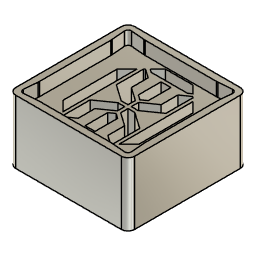
teenage_engineering_display (Autodesk Fusion 360 design; units mm, degrees)
Autodesk Fusion 360 part; units mm, degrees
sketch "8x8_led_matrix_display" plane through (0, 0, 0) normal (0, 0, 1) x (1, 0, 0)
  circle A0 centre (-14, 14) radius 1.5
  circle A1 centre (-10, 14) radius 1.5
  circle A2 centre (-6, 14) radius 1.5
  circle A3 centre (-2, 14) radius 1.5
  circle A4 centre (2, 14) radius 1.5
  circle A5 centre (6, 14) radius 1.5
  circle A6 centre (10, 14) radius 1.5
  circle A7 centre (14, 14) radius 1.5
  circle A8 centre (-14, 10) radius 1.5
  circle A9 centre (-10, 10) radius 1.5
  circle A10 centre (-6, 10) radius 1.5
  circle A11 centre (-2, 10) radius 1.5
  circle A12 centre (2, 10) radius 1.5
  circle A13 centre (6, 10) radius 1.5
  circle A14 centre (10, 10) radius 1.5
  circle A15 centre (14, 10) radius 1.5
  circle A16 centre (-14, 6) radius 1.5
  circle A17 centre (-10, 6) radius 1.5
  circle A18 centre (-6, 6) radius 1.5
  circle A19 centre (-2, 6) radius 1.5
  circle A20 centre (2, 6) radius 1.5
  circle A21 centre (6, 6) radius 1.5
  circle A22 centre (10, 6) radius 1.5
  circle A23 centre (14, 6) radius 1.5
  circle A24 centre (-14, 2) radius 1.5
  circle A25 centre (-10, 2) radius 1.5
  circle A26 centre (-6, 2) radius 1.5
  circle A27 centre (-2, 2) radius 1.5
  circle A28 centre (2, 2) radius 1.5
  circle A29 centre (6, 2) radius 1.5
  circle A30 centre (10, 2) radius 1.5
  circle A31 centre (14, 2) radius 1.5
  circle A32 centre (-14, -2) radius 1.5
  circle A33 centre (-10, -2) radius 1.5
  circle A34 centre (-6, -2) radius 1.5
  circle A35 centre (-2, -2) radius 1.5
  circle A36 centre (2, -2) radius 1.5
  circle A37 centre (6, -2) radius 1.5
  circle A38 centre (10, -2) radius 1.5
  circle A39 centre (14, -2) radius 1.5
  circle A40 centre (-14, -6) radius 1.5
  circle A41 centre (-10, -6) radius 1.5
  circle A42 centre (-6, -6) radius 1.5
  circle A43 centre (-2, -6) radius 1.5
  circle A44 centre (2, -6) radius 1.5
  circle A45 centre (6, -6) radius 1.5
  circle A46 centre (10, -6) radius 1.5
  circle A47 centre (14, -6) radius 1.5
  circle A48 centre (-14, -10) radius 1.5
  circle A49 centre (-10, -10) radius 1.5
  circle A50 centre (-6, -10) radius 1.5
  circle A51 centre (-2, -10) radius 1.5
  circle A52 centre (2, -10) radius 1.5
  circle A53 centre (6, -10) radius 1.5
  circle A54 centre (10, -10) radius 1.5
  circle A55 centre (14, -10) radius 1.5
  circle A56 centre (-14, -14) radius 1.5
  circle A57 centre (-10, -14) radius 1.5
  circle A58 centre (-6, -14) radius 1.5
  circle A59 centre (-2, -14) radius 1.5
  circle A60 centre (2, -14) radius 1.5
  circle A61 centre (6, -14) radius 1.5
  circle A62 centre (10, -14) radius 1.5
  circle A63 centre (14, -14) radius 1.5
  line L0 (16, -16) -> (-16, -16)
  line L1 (-16, -16) -> (-16, 16)
  line L2 (-16, 16) -> (16, 16)
  line L3 (16, 16) -> (16, -16)
  line L4 (16, -16) -> (-16, 16) construction
  line L5 (-16, -16) -> (16, 16) construction
  line L6 (18, -18) -> (-18, -18)
  line L7 (-18, -18) -> (-18, 18)
  line L8 (-18, 18) -> (18, 18)
  line L9 (18, 18) -> (18, -18)
  dimension "d1" = 3
  dimension "d2" = 14
  dimension "d3" = 14
  dimension "d6" = 28
  dimension "d7" = -28
  dimension "d8" = 32
  dimension "d9" = 32
  dimension "d33" = -2
  constraint horizontal L0
  constraint perpendicular L0 L1
  constraint parallel L0 L2
  constraint parallel L1 L3
  constraint coincident L4 origin
  constraint coincident L5 origin
  measures "d1" diameter of A0
  measures "d2" horizontal distance of origin A0.centre
  measures "d3" vertical distance of origin A0.centre
  measures "d8" distance of L1.end L2.end
  measures "d9" distance of L0.end L1.end
sketch "segments" plane through (0, 0, 0) normal (0, 0, 1) x (1, 0, 0)
  line L0 (0, 0) -> (-16, 0)
  line L1 (-16, 0) -> (-16, 16)
  line L2 (-16, 16) -> (0, 16)
  line L3 (0, 16) -> (0, 0)
  line L4 (-11.5, 0) -> (-11.5, 8.1712)
  line L5 (-11.5, 8.1712) -> (-8.5, 11.1712)
  line L6 (-8.5, 11.1712) -> (-8.5, 0)
  line L7 (-7.5, 12.1712) -> (-7.5, 3.961)
  line L8 (-7.5, 3.961) -> (-2.5572, 0.5)
  line L9 (-2.5572, 0.5) -> (-0.5, 0.5)
  line L10 (-0.5, 0.5) -> (-0.5, 2.7218)
  line L11 (-0.5, 2.7218) -> (-4.5, 5.5227)
  line L12 (-4.5, 5.5227) -> (-4.5, 10.5993)
  line L13 (-4.5, 10.5993) -> (-7.189, 12.4822)
  line L14 (-7.189, 12.4822) -> (-7.5, 12.1712)
  line L15 (0, 11.5) -> (-1.5, 11.5)
  line L16 (-1.5, 11.5) -> (-1.5, 4.6428)
  line L17 (-1.5, 4.6428) -> (0, 3.5925)
  line L18 (0, 15.5) -> (-4.1712, 15.5)
  line L19 (-4.1712, 15.5) -> (-6.471, 13.2002)
  line L20 (-6.471, 13.2002) -> (-5.471, 12.5)
  line L21 (-5.471, 12.5) -> (0, 12.5)
  dimension "d10" = 16
  dimension "d11" = 16
  dimension "d12" = 3
  dimension "d13" = 8.5
  dimension "d14" = 3
  dimension "d15" = 3
  dimension "d16" = 0.5
  dimension "d17" = 0.5
  dimension "d18" = 1
  dimension "d19" = 1.5
  dimension "d20" = 11.5
  dimension "d21" = 1
  dimension "d22" = 3
  dimension "d23" = 15.5
  dimension "d24" = 1
  dimension "d25" = 45
  dimension "d26" = 125
  constraint horizontal L0
  constraint vertical L1
  constraint horizontal L2
  constraint vertical L3
  constraint coincident L0.start L3.end
  constraint coincident L0 L4.start
  constraint perpendicular L0 L4
  constraint coincident L0 L6.end
  constraint perpendicular L0 L6
  constraint parallel L6 L7
  constraint perpendicular L6 L9
  constraint perpendicular L9 L10
  constraint parallel L8 L11
  constraint perpendicular L9 L12
  constraint collinear L5 L14
  constraint coincident L3 L15.start
  constraint perpendicular L3 L15
  constraint perpendicular L15 L16
  constraint coincident L3 L17.end
  constraint parallel L11 L17
  constraint coincident L3 L18.start
  constraint perpendicular L3 L18
  constraint coincident L3 L21.end
  constraint perpendicular L3 L21
  constraint parallel L13 L20
  constraint collinear L14 L19
  constraint parallel L11 L13
  measures "d10" distance of L0.start L0.end
  measures "d11" distance of L0.start L2.end
  measures "d12" distance of L4 L6
  measures "d13" distance of L3 L6
  measures "d14" distance of L7 L12
  measures "d15" distance of L8 L11
  measures "d16" distance of L3 L10
  measures "d17" distance of L0 L9
  measures "d18" distance of L6 L7
  measures "d19" distance of L3 L16
  measures "d20" distance of L0 L15
  measures "d21" distance of L11 L17
  measures "d22" distance of L18 L21
  measures "d23" distance of L0 L18
  measures "d24" distance of L13 L20
  measures "d25" angle of L5 L6
  measures "d26" angle of L12 L13
extrude "Extrude1" add sketch "segments" along normal blind 15 contours L0 L1 L2 L3 L4 L5 L6 L15 L16 L17 L18 L19 L20 L21
mirror "Mirror1" about plane through (0, 0, 0) normal (1, 0, 0) of bodies 1 merged
mirror "Mirror2" about plane through (0, 0, 0) normal (0, 1, 0) of bodies 1 merged
extrude "Extrude2" add sketch "8x8_led_matrix_display" along normal blind 15 contours L6 L7 L8 L9
fillet "Fillet1" radius 2 4 edges at (-18, -18, 7.5) (18, -18, 7.5) (18, 18, 7.5) (-18, 18, 7.5)
sketch "projected_for_diffuser" plane through (0, 0, 0) normal (0, 0, -1) x (1, 0, 0)
  arc A0 (-18, -16) -> (-16, -18) centre (-16, -16) ccw
  line L0 (-16, -18) -> (16, -18)
  arc A1 (16, -18) -> (18, -16) centre (16, -16) ccw
  line L1 (18, -16) -> (18, 16)
  arc A2 (18, 16) -> (16, 18) centre (16, 16) ccw
  line L2 (16, 18) -> (-16, 18)
  arc A3 (-16, 18) -> (-18, 16) centre (-16, 16) ccw
  line L3 (-18, 16) -> (-18, -16)
  line L4 (11.5, 8.1712) -> (11.5, -8.1712)
  line L5 (11.5, -8.1712) -> (8.5, -11.1712)
  line L6 (8.5, -11.1712) -> (8.5, 11.1712)
  line L7 (8.5, 11.1712) -> (11.5, 8.1712)
  line L8 (-7.5, 12.1712) -> (-7.189, 12.4822)
  line L9 (-7.189, 12.4822) -> (-4.5, 10.5993)
  line L10 (-4.5, 10.5993) -> (-4.5, 5.5227)
  line L11 (-4.5, 5.5227) -> (-0.5, 2.7218)
  line L12 (-0.5, 2.7218) -> (-0.5, 0.5)
  line L13 (-0.5, 0.5) -> (-2.5572, 0.5)
  line L14 (-2.5572, 0.5) -> (-7.5, 3.961)
  line L15 (-7.5, 3.961) -> (-7.5, 12.1712)
  line L16 (7.189, 12.4822) -> (7.5, 12.1712)
  line L17 (7.5, 12.1712) -> (7.5, 3.961)
  line L18 (7.5, 3.961) -> (2.5572, 0.5)
  line L19 (2.5572, 0.5) -> (0.5, 0.5)
  line L20 (0.5, 0.5) -> (0.5, 2.7218)
  line L21 (0.5, 2.7218) -> (4.5, 5.5227)
  line L22 (4.5, 5.5227) -> (4.5, 10.5993)
  line L23 (4.5, 10.5993) -> (7.189, 12.4822)
  line L24 (-1.5, 11.5) -> (1.5, 11.5)
  line L25 (1.5, 11.5) -> (1.5, 4.6428)
  line L26 (1.5, 4.6428) -> (0, 3.5925)
  line L27 (0, 3.5925) -> (-1.5, 4.6428)
  line L28 (-1.5, 4.6428) -> (-1.5, 11.5)
  line L29 (-4.1712, 15.5) -> (4.1712, 15.5)
  line L30 (4.1712, 15.5) -> (6.471, 13.2002)
  line L31 (6.471, 13.2002) -> (5.471, 12.5)
  line L32 (5.471, 12.5) -> (-5.471, 12.5)
  line L33 (-5.471, 12.5) -> (-6.471, 13.2002)
  line L34 (-6.471, 13.2002) -> (-4.1712, 15.5)
  line L35 (4.1712, -15.5) -> (-4.1712, -15.5)
  line L36 (-4.1712, -15.5) -> (-6.471, -13.2002)
  line L37 (-6.471, -13.2002) -> (-5.471, -12.5)
  line L38 (-5.471, -12.5) -> (5.471, -12.5)
  line L39 (5.471, -12.5) -> (6.471, -13.2002)
  line L40 (6.471, -13.2002) -> (4.1712, -15.5)
  line L41 (1.5, -11.5) -> (-1.5, -11.5)
  line L42 (-1.5, -11.5) -> (-1.5, -4.6428)
  line L43 (-1.5, -4.6428) -> (0, -3.5925)
  line L44 (0, -3.5925) -> (1.5, -4.6428)
  line L45 (1.5, -4.6428) -> (1.5, -11.5)
  line L46 (7.5, -12.1712) -> (7.189, -12.4822)
  line L47 (7.189, -12.4822) -> (4.5, -10.5993)
  line L48 (4.5, -10.5993) -> (4.5, -5.5227)
  line L49 (4.5, -5.5227) -> (0.5, -2.7218)
  line L50 (0.5, -2.7218) -> (0.5, -0.5)
  line L51 (0.5, -0.5) -> (2.5572, -0.5)
  line L52 (2.5572, -0.5) -> (7.5, -3.961)
  line L53 (7.5, -3.961) -> (7.5, -12.1712)
  line L54 (-7.189, -12.4822) -> (-7.5, -12.1712)
  line L55 (-7.5, -12.1712) -> (-7.5, -3.961)
  line L56 (-7.5, -3.961) -> (-2.5572, -0.5)
  line L57 (-2.5572, -0.5) -> (-0.5, -0.5)
  line L58 (-0.5, -0.5) -> (-0.5, -2.7218)
  line L59 (-0.5, -2.7218) -> (-4.5, -5.5227)
  line L60 (-4.5, -5.5227) -> (-4.5, -10.5993)
  line L61 (-4.5, -10.5993) -> (-7.189, -12.4822)
  line L62 (-11.5, -8.1712) -> (-11.5, 8.1712)
  line L63 (-11.5, 8.1712) -> (-8.5, 11.1712)
  line L64 (-8.5, 11.1712) -> (-8.5, -11.1712)
  line L65 (-8.5, -11.1712) -> (-11.5, -8.1712)
extrude "Extrude3" add sketch "projected_for_diffuser" along normal blind 0.2 contours A0 L0 A1 L1 A2 L2 A3 L3 | L4 L5 L6 L7 | L8 L9 L10 L11 L12 L13 L14 L15 | L16 L17 L18 L19 L20 L21 L22 L23 | L24 L25 L26 L27 L28 | L29 L30 L31 L32 L33 L34 | L35 L36 L37 L38 L39 L40 | L41 L42 L43 L44 L45 | L46 L47 L48 L49 L50 L51 L52 L53 | L54 L55 L56 L57 L58 L59 L60 L61 | L62 L63 L64 L65
sketch "grip_for_display" plane through (0, 0, 15) normal (0, 0, 1) x (-1, 0, 0)
  line L0 (16, -16) -> (-16, -16)
  line L1 (-16, -16) -> (-16, 16)
  line L2 (-16, 16) -> (16, 16)
  line L3 (16, 16) -> (16, -16)
  line L4 (16, -16) -> (-16, 16) construction
  line L5 (-16, -16) -> (16, 16) construction
  line L6 (16, -11) -> (-16, -11)
  line L7 (-16, -11) -> (-16, 11)
  line L8 (-16, 11) -> (16, 11)
  line L9 (16, 11) -> (16, -11)
  line L10 (16, -11) -> (-16, 11) construction
  line L11 (-16, -11) -> (16, 11) construction
  line L12 (11, -16) -> (-11, -16)
  line L13 (-11, -16) -> (-11, 16)
  line L14 (-11, 16) -> (11, 16)
  line L15 (11, 16) -> (11, -16)
  line L16 (11, -16) -> (-11, 16) construction
  line L17 (-11, -16) -> (11, 16) construction
  line L18 (-16, 11) -> (-16.4794, 16.4794)
  line L19 (-16.4794, 16.4794) -> (-11, 16)
  line L20 (11, 16) -> (16.4794, 16.4794)
  line L21 (16.4794, 16.4794) -> (16, 11)
  line L22 (16, -11) -> (16.4794, -16.4794)
  line L23 (16.4794, -16.4794) -> (11, -16)
  line L24 (-16, -11) -> (-16.4794, -16.4794)
  line L25 (-16.4794, -16.4794) -> (-11, -16)
  line L26 (-16, -18) -> (16, -18)
  arc A0 (-18, -16) -> (-16, -18) centre (-16, -16) ccw
  line L27 (-18, 16) -> (-18, -16)
  arc A1 (-16, 18) -> (-18, 16) centre (-16, 16) ccw
  line L28 (16, 18) -> (-16, 18)
  arc A2 (18, 16) -> (16, 18) centre (16, 16) ccw
  line L29 (18, -16) -> (18, 16)
  arc A3 (16, -18) -> (18, -16) centre (16, -16) ccw
  dimension "d40" = 32
  dimension "d41" = 32
  dimension "d42" = 32
  dimension "d43" = 22
  dimension "d44" = 22
  dimension "d45" = 32
  dimension "d46" = 80
  constraint horizontal L0
  constraint perpendicular L0 L1
  constraint parallel L0 L2
  constraint parallel L1 L3
  constraint coincident L4 origin
  constraint coincident L5 origin
  constraint horizontal L6
  constraint perpendicular L6 L7
  constraint parallel L6 L8
  constraint parallel L7 L9
  constraint coincident L10 origin
  constraint coincident L11 origin
  constraint horizontal L12
  constraint perpendicular L12 L13
  constraint parallel L12 L14
  constraint parallel L13 L15
  constraint coincident L16 origin
  constraint coincident L17 origin
  constraint equal L18 L19
  constraint equal L24 L25
  constraint equal L23 L25
  constraint equal L22 L23
  constraint equal L21 L22
  constraint equal L20 L21
  constraint equal L19 L20
  measures "d40" distance of L1.end L2.end
  measures "d41" distance of L0.end L1.end
  measures "d42" distance of L7.end L8.end
  measures "d43" distance of L6.end L7.end
  measures "d44" distance of L13.end L14.end
  measures "d45" distance of L12.end L13.end
  measures "d46" angle of L18 L19
extrude "Extrude4" add sketch "grip_for_display" along normal blind 4
fillet "Fillet2" radius 1 4 edges at (16.4794, -16.4794, 17) (-16.4794, -16.4794, 17) (-16.4794, 16.4794, 17) (16.4794, 16.4794, 17)
fillet "Fillet2" radius 5 8 edges at (16, -11, 17) (11, -16, 17) (-11, -16, 17) (-16, -11, 17) (-16, 11, 17) (-11, 16, 17) (11, 16, 17) (16, 11, 17)
equation "d2 = ( 3.5 * 4 ) * 1 mm"
equation "d3 = ( 3.5 * 4 ) * 1 mm"
equation "d6 = ( 4 * 7 ) * 1 mm"
equation "d7 = ( -4 * 7 ) * 1 mm"
named bodies: "teenage_engineering_display_8x8_overlay"
